Autodesk Fusion 360 part; units mm, degrees
(part 10 of 12)
  line L950 (83.2448, 72.1244) -> (83.2448, 77.1244)
  line L951 (83.2448, 77.1244) -> (78.9146, 79.6244)
  line L952 (89.5749, 79.6244) -> (85.2448, 77.1244)
  line L953 (85.2448, 77.1244) -> (85.2448, 72.1244)
  line L954 (85.2448, 72.1244) -> (89.5749, 69.6244)
  line L955 (89.5749, 69.6244) -> (93.905, 72.1244)
  line L956 (93.905, 72.1244) -> (93.905, 77.1244)
  line L957 (93.905, 77.1244) -> (89.5749, 79.6244)
  line L958 (100.2351, 79.6244) -> (95.905, 77.1244)
  line L959 (95.905, 77.1244) -> (95.905, 72.1244)
  line L960 (95.905, 72.1244) -> (100.2351, 69.6244)
  line L961 (100.2351, 69.6244) -> (104.5653, 72.1244)
  line L962 (104.5653, 72.1244) -> (104.5653, 77.1244)
  line L963 (104.5653, 77.1244) -> (100.2351, 79.6244)
  line L964 (110.8954, 79.6244) -> (106.5653, 77.1244)
  line L965 (106.5653, 77.1244) -> (106.5653, 72.1244)
  line L966 (106.5653, 72.1244) -> (110.8954, 69.6244)
  line L967 (110.8954, 69.6244) -> (115.2255, 72.1244)
  line L968 (115.2255, 72.1244) -> (115.2255, 77.1244)
  line L969 (115.2255, 77.1244) -> (110.8954, 79.6244)
  line L970 (121.5556, 79.6244) -> (117.2255, 77.1244)
  line L971 (117.2255, 77.1244) -> (117.2255, 72.1244)
  line L972 (117.2255, 72.1244) -> (121.5556, 69.6244)
  line L973 (121.5556, 69.6244) -> (125.8858, 72.1244)
  line L974 (125.8858, 72.1244) -> (125.8858, 77.1244)
  line L975 (125.8858, 77.1244) -> (121.5556, 79.6244)
  line L976 (132.2159, 79.6244) -> (127.8858, 77.1244)
  line L977 (127.8858, 77.1244) -> (127.8858, 72.1244)
  line L978 (127.8858, 72.1244) -> (132.2159, 69.6244)
  line L979 (132.2159, 69.6244) -> (136.546, 72.1244)
  line L980 (136.546, 72.1244) -> (136.546, 77.1244)
  line L981 (136.546, 77.1244) -> (132.2159, 79.6244)
  line L982 (142.8762, 79.6244) -> (138.546, 77.1244)
  line L983 (138.546, 77.1244) -> (138.546, 72.1244)
  line L984 (138.546, 72.1244) -> (142.8762, 69.6244)
  line L985 (142.8762, 69.6244) -> (147.2063, 72.1244)
  line L986 (147.2063, 72.1244) -> (147.2063, 77.1244)
  line L987 (147.2063, 77.1244) -> (142.8762, 79.6244)
  line L988 (-64.9988, 88.8564) -> (-69.3289, 86.3564)
  line L989 (-69.3289, 86.3564) -> (-69.3289, 81.3564)
  line L990 (-69.3289, 81.3564) -> (-64.9988, 78.8564)
  line L991 (-64.9988, 78.8564) -> (-60.6687, 81.3564)
  line L992 (-60.6687, 81.3564) -> (-60.6687, 86.3564)
  line L993 (-60.6687, 86.3564) -> (-64.9988, 88.8564)
  line L994 (-54.3385, 88.8564) -> (-58.6687, 86.3564)
  line L995 (-58.6687, 86.3564) -> (-58.6687, 81.3564)
  line L996 (-58.6687, 81.3564) -> (-54.3385, 78.8564)
  line L997 (-54.3385, 78.8564) -> (-50.0084, 81.3564)
  line L998 (-50.0084, 81.3564) -> (-50.0084, 86.3564)
  line L999 (-50.0084, 86.3564) -> (-54.3385, 88.8564)
  line L1000 (-43.6783, 88.8564) -> (-48.0084, 86.3564)
  line L1001 (-48.0084, 86.3564) -> (-48.0084, 81.3564)
  line L1002 (-48.0084, 81.3564) -> (-43.6783, 78.8564)
  line L1003 (-43.6783, 78.8564) -> (-39.3482, 81.3564)
  line L1004 (-39.3482, 81.3564) -> (-39.3482, 86.3564)
  line L1005 (-39.3482, 86.3564) -> (-43.6783, 88.8564)
  line L1006 (-33.018, 88.8564) -> (-37.3482, 86.3564)
  line L1007 (-37.3482, 86.3564) -> (-37.3482, 81.3564)
  line L1008 (-37.3482, 81.3564) -> (-33.018, 78.8564)
  line L1009 (-33.018, 78.8564) -> (-28.6879, 81.3564)
  line L1010 (-28.6879, 81.3564) -> (-28.6879, 86.3564)
  line L1011 (-28.6879, 86.3564) -> (-33.018, 88.8564)
  line L1012 (-22.3578, 88.8564) -> (-26.6879, 86.3564)
  line L1013 (-26.6879, 86.3564) -> (-26.6879, 81.3564)
  line L1014 (-26.6879, 81.3564) -> (-22.3578, 78.8564)
  line L1015 (-22.3578, 78.8564) -> (-18.0277, 81.3564)
  line L1016 (-18.0277, 81.3564) -> (-18.0277, 86.3564)
  line L1017 (-18.0277, 86.3564) -> (-22.3578, 88.8564)
  line L1018 (-11.6975, 88.8564) -> (-16.0277, 86.3564)
  line L1019 (-16.0277, 86.3564) -> (-16.0277, 81.3564)
  line L1020 (-16.0277, 81.3564) -> (-11.6975, 78.8564)
  line L1021 (-11.6975, 78.8564) -> (-7.3674, 81.3564)
  line L1022 (-7.3674, 81.3564) -> (-7.3674, 86.3564)
  line L1023 (-7.3674, 86.3564) -> (-11.6975, 88.8564)
  line L1024 (-1.0373, 88.8564) -> (-5.3674, 86.3564)
  line L1025 (-5.3674, 86.3564) -> (-5.3674, 81.3564)
  line L1026 (-5.3674, 81.3564) -> (-1.0373, 78.8564)
  line L1027 (-1.0373, 78.8564) -> (3.2929, 81.3564)
  line L1028 (3.2929, 81.3564) -> (3.2929, 86.3564)
  line L1029 (3.2929, 86.3564) -> (-1.0373, 88.8564)
  line L1030 (9.623, 88.8564) -> (5.2929, 86.3564)
  line L1031 (5.2929, 86.3564) -> (5.2929, 81.3564)
  line L1032 (5.2929, 81.3564) -> (9.623, 78.8564)
  line L1033 (9.623, 78.8564) -> (13.9531, 81.3564)
  line L1034 (13.9531, 81.3564) -> (13.9531, 86.3564)
  line L1035 (13.9531, 86.3564) -> (9.623, 88.8564)
  line L1036 (20.2832, 88.8564) -> (15.9531, 86.3564)
  line L1037 (15.9531, 86.3564) -> (15.9531, 81.3564)
  line L1038 (15.9531, 81.3564) -> (20.2832, 78.8564)
  line L1039 (20.2832, 78.8564) -> (24.6134, 81.3564)
  line L1040 (24.6134, 81.3564) -> (24.6134, 86.3564)
  line L1041 (24.6134, 86.3564) -> (20.2832, 88.8564)
  line L1042 (30.9435, 88.8564) -> (26.6134, 86.3564)
  line L1043 (26.6134, 86.3564) -> (26.6134, 81.3564)
  line L1044 (26.6134, 81.3564) -> (30.9435, 78.8564)
  line L1045 (30.9435, 78.8564) -> (35.2736, 81.3564)
  line L1046 (35.2736, 81.3564) -> (35.2736, 86.3564)
  line L1047 (35.2736, 86.3564) -> (30.9435, 88.8564)
  line L1048 (41.6037, 88.8564) -> (37.2736, 86.3564)
  line L1049 (37.2736, 86.3564) -> (37.2736, 81.3564)
  line L1050 (37.2736, 81.3564) -> (41.6037, 78.8564)
  line L1051 (41.6037, 78.8564) -> (45.9339, 81.3564)
  line L1052 (45.9339, 81.3564) -> (45.9339, 86.3564)
  line L1053 (45.9339, 86.3564) -> (41.6037, 88.8564)
  line L1054 (52.264, 88.8564) -> (47.9339, 86.3564)
  line L1055 (47.9339, 86.3564) -> (47.9339, 81.3564)
  line L1056 (47.9339, 81.3564) -> (52.264, 78.8564)
  line L1057 (52.264, 78.8564) -> (56.5941, 81.3564)
  line L1058 (56.5941, 81.3564) -> (56.5941, 86.3564)
  line L1059 (56.5941, 86.3564) -> (52.264, 88.8564)
  line L1060 (62.9242, 88.8564) -> (58.5941, 86.3564)
  line L1061 (58.5941, 86.3564) -> (58.5941, 81.3564)
  line L1062 (58.5941, 81.3564) -> (62.9242, 78.8564)
  line L1063 (62.9242, 78.8564) -> (67.2544, 81.3564)
  line L1064 (67.2544, 81.3564) -> (67.2544, 86.3564)
  line L1065 (67.2544, 86.3564) -> (62.9242, 88.8564)
  line L1066 (73.5845, 88.8564) -> (69.2544, 86.3564)
  line L1067 (69.2544, 86.3564) -> (69.2544, 81.3564)
  line L1068 (69.2544, 81.3564) -> (73.5845, 78.8564)
  line L1069 (73.5845, 78.8564) -> (77.9146, 81.3564)
  line L1070 (77.9146, 81.3564) -> (77.9146, 86.3564)
  line L1071 (77.9146, 86.3564) -> (73.5845, 88.8564)
  line L1072 (84.2448, 88.8564) -> (79.9146, 86.3564)
  line L1073 (79.9146, 86.3564) -> (79.9146, 81.3564)
  line L1074 (79.9146, 81.3564) -> (84.2448, 78.8564)
  line L1075 (84.2448, 78.8564) -> (88.5749, 81.3564)
  line L1076 (88.5749, 81.3564) -> (88.5749, 86.3564)
  line L1077 (88.5749, 86.3564) -> (84.2448, 88.8564)
  line L1078 (94.905, 88.8564) -> (90.5749, 86.3564)
  line L1079 (90.5749, 86.3564) -> (90.5749, 81.3564)
  line L1080 (90.5749, 81.3564) -> (94.905, 78.8564)
  line L1081 (94.905, 78.8564) -> (99.2351, 81.3564)
  line L1082 (99.2351, 81.3564) -> (99.2351, 86.3564)
  line L1083 (99.2351, 86.3564) -> (94.905, 88.8564)
  line L1084 (105.5653, 88.8564) -> (101.2351, 86.3564)
  line L1085 (101.2351, 86.3564) -> (101.2351, 81.3564)
  line L1086 (101.2351, 81.3564) -> (105.5653, 78.8564)
  line L1087 (105.5653, 78.8564) -> (109.8954, 81.3564)
  line L1088 (109.8954, 81.3564) -> (109.8954, 86.3564)
  line L1089 (109.8954, 86.3564) -> (105.5653, 88.8564)
  line L1090 (116.2255, 88.8564) -> (111.8954, 86.3564)
  line L1091 (111.8954, 86.3564) -> (111.8954, 81.3564)
  line L1092 (111.8954, 81.3564) -> (116.2255, 78.8564)
  line L1093 (116.2255, 78.8564) -> (120.5556, 81.3564)
  line L1094 (120.5556, 81.3564) -> (120.5556, 86.3564)
  line L1095 (120.5556, 86.3564) -> (116.2255, 88.8564)
  line L1096 (126.8858, 88.8564) -> (122.5556, 86.3564)
  line L1097 (122.5556, 86.3564) -> (122.5556, 81.3564)
  line L1098 (122.5556, 81.3564) -> (126.8858, 78.8564)
  line L1099 (126.8858, 78.8564) -> (131.2159, 81.3564)
  line L1100 (131.2159, 81.3564) -> (131.2159, 86.3564)
  line L1101 (131.2159, 86.3564) -> (126.8858, 88.8564)
  line L1102 (137.546, 88.8564) -> (133.2159, 86.3564)
  line L1103 (133.2159, 86.3564) -> (133.2159, 81.3564)
  line L1104 (133.2159, 81.3564) -> (137.546, 78.8564)
  line L1105 (137.546, 78.8564) -> (141.8762, 81.3564)
  line L1106 (141.8762, 81.3564) -> (141.8762, 86.3564)
  line L1107 (141.8762, 86.3564) -> (137.546, 88.8564)
  line L1108 (148.2063, 88.8564) -> (143.8762, 86.3564)
  line L1109 (143.8762, 86.3564) -> (143.8762, 81.3564)
  line L1110 (143.8762, 81.3564) -> (148.2063, 78.8564)
  line L1111 (148.2063, 78.8564) -> (152.5364, 81.3564)
  line L1112 (152.5364, 81.3564) -> (152.5364, 86.3564)
  line L1113 (152.5364, 86.3564) -> (148.2063, 88.8564)
  line L1114 (-59.6687, 98.0885) -> (-63.9988, 95.5885)
  line L1115 (-63.9988, 95.5885) -> (-63.9988, 90.5885)
  line L1116 (-63.9988, 90.5885) -> (-59.6687, 88.0885)
  line L1117 (-59.6687, 88.0885) -> (-55.3385, 90.5885)
  line L1118 (-55.3385, 90.5885) -> (-55.3385, 95.5885)
  line L1119 (-55.3385, 95.5885) -> (-59.6687, 98.0885)
  line L1120 (-49.0084, 98.0885) -> (-53.3385, 95.5885)
  line L1121 (-53.3385, 95.5885) -> (-53.3385, 90.5885)
  line L1122 (-53.3385, 90.5885) -> (-49.0084, 88.0885)
  line L1123 (-49.0084, 88.0885) -> (-44.6783, 90.5885)
  line L1124 (-44.6783, 90.5885) -> (-44.6783, 95.5885)
  line L1125 (-44.6783, 95.5885) -> (-49.0084, 98.0885)
  line L1126 (-38.3482, 98.0885) -> (-42.6783, 95.5885)
  line L1127 (-42.6783, 95.5885) -> (-42.6783, 90.5885)
  line L1128 (-42.6783, 90.5885) -> (-38.3482, 88.0885)
  line L1129 (-38.3482, 88.0885) -> (-34.018, 90.5885)
  line L1130 (-34.018, 90.5885) -> (-34.018, 95.5885)
  line L1131 (-34.018, 95.5885) -> (-38.3482, 98.0885)
  line L1132 (-27.6879, 98.0885) -> (-32.018, 95.5885)
  line L1133 (-32.018, 95.5885) -> (-32.018, 90.5885)
  line L1134 (-32.018, 90.5885) -> (-27.6879, 88.0885)
  line L1135 (-27.6879, 88.0885) -> (-23.3578, 90.5885)
  line L1136 (-23.3578, 90.5885) -> (-23.3578, 95.5885)
  line L1137 (-23.3578, 95.5885) -> (-27.6879, 98.0885)
  line L1138 (-17.0277, 98.0885) -> (-21.3578, 95.5885)
  line L1139 (-21.3578, 95.5885) -> (-21.3578, 90.5885)
  line L1140 (-21.3578, 90.5885) -> (-17.0277, 88.0885)
  line L1141 (-17.0277, 88.0885) -> (-12.6975, 90.5885)
  line L1142 (-12.6975, 90.5885) -> (-12.6975, 95.5885)
  line L1143 (-12.6975, 95.5885) -> (-17.0277, 98.0885)
  line L1144 (-6.3674, 98.0885) -> (-10.6975, 95.5885)
  line L1145 (-10.6975, 95.5885) -> (-10.6975, 90.5885)
  line L1146 (-10.6975, 90.5885) -> (-6.3674, 88.0885)
  line L1147 (-6.3674, 88.0885) -> (-2.0373, 90.5885)
  line L1148 (-2.0373, 90.5885) -> (-2.0373, 95.5885)
  line L1149 (-2.0373, 95.5885) -> (-6.3674, 98.0885)
  line L1150 (4.2929, 98.0885) -> (-0.0373, 95.5885)
  line L1151 (-0.0373, 95.5885) -> (-0.0373, 90.5885)
  line L1152 (-0.0373, 90.5885) -> (4.2929, 88.0885)
  line L1153 (4.2929, 88.0885) -> (8.623, 90.5885)
  line L1154 (8.623, 90.5885) -> (8.623, 95.5885)
  line L1155 (8.623, 95.5885) -> (4.2929, 98.0885)
  line L1156 (14.9531, 98.0885) -> (10.623, 95.5885)
  line L1157 (10.623, 95.5885) -> (10.623, 90.5885)
  line L1158 (10.623, 90.5885) -> (14.9531, 88.0885)
  line L1159 (14.9531, 88.0885) -> (19.2832, 90.5885)
  line L1160 (19.2832, 90.5885) -> (19.2832, 95.5885)
  line L1161 (19.2832, 95.5885) -> (14.9531, 98.0885)
  line L1162 (25.6134, 98.0885) -> (21.2832, 95.5885)
  line L1163 (21.2832, 95.5885) -> (21.2832, 90.5885)
  line L1164 (21.2832, 90.5885) -> (25.6134, 88.0885)
  line L1165 (25.6134, 88.0885) -> (29.9435, 90.5885)
  line L1166 (29.9435, 90.5885) -> (29.9435, 95.5885)
  line L1167 (29.9435, 95.5885) -> (25.6134, 98.0885)
  line L1168 (36.2736, 98.0885) -> (31.9435, 95.5885)
  line L1169 (31.9435, 95.5885) -> (31.9435, 90.5885)
  line L1170 (31.9435, 90.5885) -> (36.2736, 88.0885)
  line L1171 (36.2736, 88.0885) -> (40.6037, 90.5885)
  line L1172 (40.6037, 90.5885) -> (40.6037, 95.5885)
  line L1173 (40.6037, 95.5885) -> (36.2736, 98.0885)
  line L1174 (46.9339, 98.0885) -> (42.6037, 95.5885)
  line L1175 (42.6037, 95.5885) -> (42.6037, 90.5885)
  line L1176 (42.6037, 90.5885) -> (46.9339, 88.0885)
  line L1177 (46.9339, 88.0885) -> (51.264, 90.5885)
  line L1178 (51.264, 90.5885) -> (51.264, 95.5885)
  line L1179 (51.264, 95.5885) -> (46.9339, 98.0885)
  line L1180 (57.5941, 98.0885) -> (53.264, 95.5885)
  line L1181 (53.264, 95.5885) -> (53.264, 90.5885)
  line L1182 (53.264, 90.5885) -> (57.5941, 88.0885)
  line L1183 (57.5941, 88.0885) -> (61.9242, 90.5885)
  line L1184 (61.9242, 90.5885) -> (61.9242, 95.5885)
  line L1185 (61.9242, 95.5885) -> (57.5941, 98.0885)
  line L1186 (68.2544, 98.0885) -> (63.9242, 95.5885)
  line L1187 (63.9242, 95.5885) -> (63.9242, 90.5885)
  line L1188 (63.9242, 90.5885) -> (68.2544, 88.0885)
  line L1189 (68.2544, 88.0885) -> (72.5845, 90.5885)
  line L1190 (72.5845, 90.5885) -> (72.5845, 95.5885)
  line L1191 (72.5845, 95.5885) -> (68.2544, 98.0885)
  line L1192 (78.9146, 98.0885) -> (74.5845, 95.5885)
  line L1193 (74.5845, 95.5885) -> (74.5845, 90.5885)
  line L1194 (74.5845, 90.5885) -> (78.9146, 88.0885)
  line L1195 (78.9146, 88.0885) -> (83.2448, 90.5885)
  line L1196 (83.2448, 90.5885) -> (83.2448, 95.5885)
  line L1197 (83.2448, 95.5885) -> (78.9146, 98.0885)
  line L1198 (89.5749, 98.0885) -> (85.2448, 95.5885)
  line L1199 (85.2448, 95.5885) -> (85.2448, 90.5885)
  line L1200 (85.2448, 90.5885) -> (89.5749, 88.0885)
  line L1201 (89.5749, 88.0885) -> (93.905, 90.5885)
  line L1202 (93.905, 90.5885) -> (93.905, 95.5885)
  line L1203 (93.905, 95.5885) -> (89.5749, 98.0885)
  line L1204 (100.2351, 98.0885) -> (95.905, 95.5885)
  line L1205 (95.905, 95.5885) -> (95.905, 90.5885)
  line L1206 (95.905, 90.5885) -> (100.2351, 88.0885)
  line L1207 (100.2351, 88.0885) -> (104.5653, 90.5885)
  line L1208 (104.5653, 90.5885) -> (104.5653, 95.5885)
  line L1209 (104.5653, 95.5885) -> (100.2351, 98.0885)
  line L1210 (110.8954, 98.0885) -> (106.5653, 95.5885)
  line L1211 (106.5653, 95.5885) -> (106.5653, 90.5885)
  line L1212 (106.5653, 90.5885) -> (110.8954, 88.0885)
  line L1213 (110.8954, 88.0885) -> (115.2255, 90.5885)
  line L1214 (115.2255, 90.5885) -> (115.2255, 95.5885)
  line L1215 (115.2255, 95.5885) -> (110.8954, 98.0885)
  line L1216 (121.5556, 98.0885) -> (117.2255, 95.5885)
  line L1217 (117.2255, 95.5885) -> (117.2255, 90.5885)
  line L1218 (117.2255, 90.5885) -> (121.5556, 88.0885)
  line L1219 (121.5556, 88.0885) -> (125.8858, 90.5885)
  line L1220 (125.8858, 90.5885) -> (125.8858, 95.5885)
  line L1221 (125.8858, 95.5885) -> (121.5556, 98.0885)
  line L1222 (132.2159, 98.0885) -> (127.8858, 95.5885)
  line L1223 (127.8858, 95.5885) -> (127.8858, 90.5885)
  line L1224 (127.8858, 90.5885) -> (132.2159, 88.0885)
  line L1225 (132.2159, 88.0885) -> (136.546, 90.5885)
  line L1226 (136.546, 90.5885) -> (136.546, 95.5885)
  line L1227 (136.546, 95.5885) -> (132.2159, 98.0885)
  line L1228 (142.8762, 98.0885) -> (138.546, 95.5885)
  line L1229 (138.546, 95.5885) -> (138.546, 90.5885)
  line L1230 (138.546, 90.5885) -> (142.8762, 88.0885)
  line L1231 (142.8762, 88.0885) -> (147.2063, 90.5885)
  line L1232 (147.2063, 90.5885) -> (147.2063, 95.5885)
  line L1233 (147.2063, 95.5885) -> (142.8762, 98.0885)
  line L1234 (-64.9988, 107.3205) -> (-69.3289, 104.8205)
  line L1235 (-69.3289, 104.8205) -> (-69.3289, 99.8205)
  line L1236 (-69.3289, 99.8205) -> (-64.9988, 97.3205)
  line L1237 (-64.9988, 97.3205) -> (-60.6687, 99.8205)
  line L1238 (-60.6687, 99.8205) -> (-60.6687, 104.8205)
  line L1239 (-60.6687, 104.8205) -> (-64.9988, 107.3205)
  line L1240 (-54.3385, 107.3205) -> (-58.6687, 104.8205)
  line L1241 (-58.6687, 104.8205) -> (-58.6687, 99.8205)
  line L1242 (-58.6687, 99.8205) -> (-54.3385, 97.3205)
  line L1243 (-54.3385, 97.3205) -> (-50.0084, 99.8205)
  line L1244 (-50.0084, 99.8205) -> (-50.0084, 104.8205)
  line L1245 (-50.0084, 104.8205) -> (-54.3385, 107.3205)
  line L1246 (-43.6783, 107.3205) -> (-48.0084, 104.8205)
  line L1247 (-48.0084, 104.8205) -> (-48.0084, 99.8205)
  line L1248 (-48.0084, 99.8205) -> (-43.6783, 97.3205)
  line L1249 (-43.6783, 97.3205) -> (-39.3482, 99.8205)
  line L1250 (-39.3482, 99.8205) -> (-39.3482, 104.8205)
  line L1251 (-39.3482, 104.8205) -> (-43.6783, 107.3205)
  line L1252 (-33.018, 107.3205) -> (-37.3482, 104.8205)
  line L1253 (-37.3482, 104.8205) -> (-37.3482, 99.8205)
  line L1254 (-37.3482, 99.8205) -> (-33.018, 97.3205)
  line L1255 (-33.018, 97.3205) -> (-28.6879, 99.8205)
  line L1256 (-28.6879, 99.8205) -> (-28.6879, 104.8205)
  line L1257 (-28.6879, 104.8205) -> (-33.018, 107.3205)
  line L1258 (-22.3578, 107.3205) -> (-26.6879, 104.8205)
  line L1259 (-26.6879, 104.8205) -> (-26.6879, 99.8205)
  line L1260 (-26.6879, 99.8205) -> (-22.3578, 97.3205)
  line L1261 (-22.3578, 97.3205) -> (-18.0277, 99.8205)
  line L1262 (-18.0277, 99.8205) -> (-18.0277, 104.8205)
  line L1263 (-18.0277, 104.8205) -> (-22.3578, 107.3205)
  line L1264 (-11.6975, 107.3205) -> (-16.0277, 104.8205)
  line L1265 (-16.0277, 104.8205) -> (-16.0277, 99.8205)
  line L1266 (-16.0277, 99.8205) -> (-11.6975, 97.3205)
  line L1267 (-11.6975, 97.3205) -> (-7.3674, 99.8205)
  line L1268 (-7.3674, 99.8205) -> (-7.3674, 104.8205)
  line L1269 (-7.3674, 104.8205) -> (-11.6975, 107.3205)
  line L1270 (-1.0373, 107.3205) -> (-5.3674, 104.8205)
  line L1271 (-5.3674, 104.8205) -> (-5.3674, 99.8205)
  line L1272 (-5.3674, 99.8205) -> (-1.0373, 97.3205)
  line L1273 (-1.0373, 97.3205) -> (3.2929, 99.8205)
  line L1274 (3.2929, 99.8205) -> (3.2929, 104.8205)
  line L1275 (3.2929, 104.8205) -> (-1.0373, 107.3205)
  line L1276 (9.623, 107.3205) -> (5.2929, 104.8205)
  line L1277 (5.2929, 104.8205) -> (5.2929, 99.8205)
  line L1278 (5.2929, 99.8205) -> (9.623, 97.3205)
  line L1279 (9.623, 97.3205) -> (13.9531, 99.8205)
  line L1280 (13.9531, 99.8205) -> (13.9531, 104.8205)
  line L1281 (13.9531, 104.8205) -> (9.623, 107.3205)
  line L1282 (20.2832, 107.3205) -> (15.9531, 104.8205)
  line L1283 (15.9531, 104.8205) -> (15.9531, 99.8205)
  line L1284 (15.9531, 99.8205) -> (20.2832, 97.3205)
  line L1285 (20.2832, 97.3205) -> (24.6134, 99.8205)
  line L1286 (24.6134, 99.8205) -> (24.6134, 104.8205)
  line L1287 (24.6134, 104.8205) -> (20.2832, 107.3205)
  line L1288 (30.9435, 107.3205) -> (26.6134, 104.8205)
  line L1289 (26.6134, 104.8205) -> (26.6134, 99.8205)
  line L1290 (26.6134, 99.8205) -> (30.9435, 97.3205)
  line L1291 (30.9435, 97.3205) -> (35.2736, 99.8205)
  line L1292 (35.2736, 99.8205) -> (35.2736, 104.8205)
  line L1293 (35.2736, 104.8205) -> (30.9435, 107.3205)
  line L1294 (41.6037, 107.3205) -> (37.2736, 104.8205)
  line L1295 (37.2736, 104.8205) -> (37.2736, 99.8205)
  line L1296 (37.2736, 99.8205) -> (41.6037, 97.3205)
  line L1297 (41.6037, 97.3205) -> (45.9339, 99.8205)
  line L1298 (45.9339, 99.8205) -> (45.9339, 104.8205)
  line L1299 (45.9339, 104.8205) -> (41.6037, 107.3205)
  line L1300 (52.264, 107.3205) -> (47.9339, 104.8205)
  line L1301 (47.9339, 104.8205) -> (47.9339, 99.8205)
  line L1302 (47.9339, 99.8205) -> (52.264, 97.3205)
  line L1303 (52.264, 97.3205) -> (56.5941, 99.8205)
  line L1304 (56.5941, 99.8205) -> (56.5941, 104.8205)
  line L1305 (56.5941, 104.8205) -> (52.264, 107.3205)
  line L1306 (62.9242, 107.3205) -> (58.5941, 104.8205)
  line L1307 (58.5941, 104.8205) -> (58.5941, 99.8205)
  line L1308 (58.5941, 99.8205) -> (62.9242, 97.3205)
  line L1309 (62.9242, 97.3205) -> (67.2544, 99.8205)
  line L1310 (67.2544, 99.8205) -> (67.2544, 104.8205)
  line L1311 (67.2544, 104.8205) -> (62.9242, 107.3205)
  line L1312 (73.5845, 107.3205) -> (69.2544, 104.8205)
  line L1313 (69.2544, 104.8205) -> (69.2544, 99.8205)
  line L1314 (69.2544, 99.8205) -> (73.5845, 97.3205)
  line L1315 (73.5845, 97.3205) -> (77.9146, 99.8205)
  line L1316 (77.9146, 99.8205) -> (77.9146, 104.8205)
  line L1317 (77.9146, 104.8205) -> (73.5845, 107.3205)
  line L1318 (84.2448, 107.3205) -> (79.9146, 104.8205)
  line L1319 (79.9146, 104.8205) -> (79.9146, 99.8205)
  line L1320 (79.9146, 99.8205) -> (84.2448, 97.3205)
  line L1321 (84.2448, 97.3205) -> (88.5749, 99.8205)
  line L1322 (88.5749, 99.8205) -> (88.5749, 104.8205)
  line L1323 (88.5749, 104.8205) -> (84.2448, 107.3205)
  line L1324 (94.905, 107.3205) -> (90.5749, 104.8205)
  line L1325 (90.5749, 104.8205) -> (90.5749, 99.8205)
  line L1326 (90.5749, 99.8205) -> (94.905, 97.3205)
  line L1327 (94.905, 97.3205) -> (99.2351, 99.8205)
  line L1328 (99.2351, 99.8205) -> (99.2351, 104.8205)
  line L1329 (99.2351, 104.8205) -> (94.905, 107.3205)
  line L1330 (105.5653, 107.3205) -> (101.2351, 104.8205)
  line L1331 (101.2351, 104.8205) -> (101.2351, 99.8205)
  line L1332 (101.2351, 99.8205) -> (105.5653, 97.3205)
  line L1333 (105.5653, 97.3205) -> (109.8954, 99.8205)
  line L1334 (109.8954, 99.8205) -> (109.8954, 104.8205)
  line L1335 (109.8954, 104.8205) -> (105.5653, 107.3205)
  line L1336 (116.2255, 107.3205) -> (111.8954, 104.8205)
  line L1337 (111.8954, 104.8205) -> (111.8954, 99.8205)
  line L1338 (111.8954, 99.8205) -> (116.2255, 97.3205)
  line L1339 (116.2255, 97.3205) -> (120.5556, 99.8205)
  line L1340 (120.5556, 99.8205) -> (120.5556, 104.8205)
  line L1341 (120.5556, 104.8205) -> (116.2255, 107.3205)
  line L1342 (126.8858, 107.3205) -> (122.5556, 104.8205)
  line L1343 (122.5556, 104.8205) -> (122.5556, 99.8205)
  line L1344 (122.5556, 99.8205) -> (126.8858, 97.3205)
  line L1345 (126.8858, 97.3205) -> (131.2159, 99.8205)
  line L1346 (131.2159, 99.8205) -> (131.2159, 104.8205)
  line L1347 (131.2159, 104.8205) -> (126.8858, 107.3205)
  line L1348 (137.546, 107.3205) -> (133.2159, 104.8205)
  line L1349 (133.2159, 104.8205) -> (133.2159, 99.8205)
  line L1350 (133.2159, 99.8205) -> (137.546, 97.3205)
  line L1351 (137.546, 97.3205) -> (141.8762, 99.8205)
  line L1352 (141.8762, 99.8205) -> (141.8762, 104.8205)
  line L1353 (141.8762, 104.8205) -> (137.546, 107.3205)
  line L1354 (148.2063, 107.3205) -> (143.8762, 104.8205)
  line L1355 (143.8762, 104.8205) -> (143.8762, 99.8205)
  line L1356 (143.8762, 99.8205) -> (148.2063, 97.3205)
  line L1357 (148.2063, 97.3205) -> (152.5364, 99.8205)
  line L1358 (152.5364, 99.8205) -> (152.5364, 104.8205)
  line L1359 (152.5364, 104.8205) -> (148.2063, 107.3205)
  line L1360 (-59.6687, 116.5526) -> (-63.9988, 114.0526)
  line L1361 (-63.9988, 114.0526) -> (-63.9988, 109.0526)
  line L1362 (-63.9988, 109.0526) -> (-59.6687, 106.5526)
  line L1363 (-59.6687, 106.5526) -> (-55.3385, 109.0526)
  line L1364 (-55.3385, 109.0526) -> (-55.3385, 114.0526)
  line L1365 (-55.3385, 114.0526) -> (-59.6687, 116.5526)
  line L1366 (-49.0084, 116.5526) -> (-53.3385, 114.0526)
  line L1367 (-53.3385, 114.0526) -> (-53.3385, 109.0526)
  line L1368 (-53.3385, 109.0526) -> (-49.0084, 106.5526)
  line L1369 (-49.0084, 106.5526) -> (-44.6783, 109.0526)
  line L1370 (-44.6783, 109.0526) -> (-44.6783, 114.0526)
  line L1371 (-44.6783, 114.0526) -> (-49.0084, 116.5526)
  line L1372 (-38.3482, 116.5526) -> (-42.6783, 114.0526)
  line L1373 (-42.6783, 114.0526) -> (-42.6783, 109.0526)
  line L1374 (-42.6783, 109.0526) -> (-38.3482, 106.5526)
  line L1375 (-38.3482, 106.5526) -> (-34.018, 109.0526)
  line L1376 (-34.018, 109.0526) -> (-34.018, 114.0526)
  line L1377 (-34.018, 114.0526) -> (-38.3482, 116.5526)
  line L1378 (-27.6879, 116.5526) -> (-32.018, 114.0526)
  line L1379 (-32.018, 114.0526) -> (-32.018, 109.0526)
  line L1380 (-32.018, 109.0526) -> (-27.6879, 106.5526)
  line L1381 (-27.6879, 106.5526) -> (-23.3578, 109.0526)
  line L1382 (-23.3578, 109.0526) -> (-23.3578, 114.0526)
  line L1383 (-23.3578, 114.0526) -> (-27.6879, 116.5526)
  line L1384 (-17.0277, 116.5526) -> (-21.3578, 114.0526)
  line L1385 (-21.3578, 114.0526) -> (-21.3578, 109.0526)
  line L1386 (-21.3578, 109.0526) -> (-17.0277, 106.5526)
  line L1387 (-17.0277, 106.5526) -> (-12.6975, 109.0526)
  line L1388 (-12.6975, 109.0526) -> (-12.6975, 114.0526)
  line L1389 (-12.6975, 114.0526) -> (-17.0277, 116.5526)
  line L1390 (-6.3674, 116.5526) -> (-10.6975, 114.0526)
  line L1391 (-10.6975, 114.0526) -> (-10.6975, 109.0526)
  line L1392 (-10.6975, 109.0526) -> (-6.3674, 106.5526)
  line L1393 (-6.3674, 106.5526) -> (-2.0373, 109.0526)
  line L1394 (-2.0373, 109.0526) -> (-2.0373, 114.0526)
  line L1395 (-2.0373, 114.0526) -> (-6.3674, 116.5526)
  line L1396 (4.2929, 116.5526) -> (-0.0373, 114.0526)
  line L1397 (-0.0373, 114.0526) -> (-0.0373, 109.0526)
  line L1398 (-0.0373, 109.0526) -> (4.2929, 106.5526)
  line L1399 (4.2929, 106.5526) -> (8.623, 109.0526)
  line L1400 (8.623, 109.0526) -> (8.623, 114.0526)
  line L1401 (8.623, 114.0526) -> (4.2929, 116.5526)
  line L1402 (14.9531, 116.5526) -> (10.623, 114.0526)
  line L1403 (10.623, 114.0526) -> (10.623, 109.0526)
  line L1404 (10.623, 109.0526) -> (14.9531, 106.5526)
  line L1405 (14.9531, 106.5526) -> (19.2832, 109.0526)
  line L1406 (19.2832, 109.0526) -> (19.2832, 114.0526)
  line L1407 (19.2832, 114.0526) -> (14.9531, 116.5526)
  line L1408 (25.6134, 116.5526) -> (21.2832, 114.0526)
  line L1409 (21.2832, 114.0526) -> (21.2832, 109.0526)
  line L1410 (21.2832, 109.0526) -> (25.6134, 106.5526)
  line L1411 (25.6134, 106.5526) -> (29.9435, 109.0526)
  line L1412 (29.9435, 109.0526) -> (29.9435, 114.0526)
  line L1413 (29.9435, 114.0526) -> (25.6134, 116.5526)
  line L1414 (36.2736, 116.5526) -> (31.9435, 114.0526)
  line L1415 (31.9435, 114.0526) -> (31.9435, 109.0526)
  line L1416 (31.9435, 109.0526) -> (36.2736, 106.5526)
  line L1417 (36.2736, 106.5526) -> (40.6037, 109.0526)
  line L1418 (40.6037, 109.0526) -> (40.6037, 114.0526)
  line L1419 (40.6037, 114.0526) -> (36.2736, 116.5526)
  line L1420 (46.9339, 116.5526) -> (42.6037, 114.0526)
  line L1421 (42.6037, 114.0526) -> (42.6037, 109.0526)
  line L1422 (42.6037, 109.0526) -> (46.9339, 106.5526)
  line L1423 (46.9339, 106.5526) -> (51.264, 109.0526)
  line L1424 (51.264, 109.0526) -> (51.264, 114.0526)
  line L1425 (51.264, 114.0526) -> (46.9339, 116.5526)
  line L1426 (57.5941, 116.5526) -> (53.264, 114.0526)
  line L1427 (53.264, 114.0526) -> (53.264, 109.0526)
  line L1428 (53.264, 109.0526) -> (57.5941, 106.5526)
  line L1429 (57.5941, 106.5526) -> (61.9242, 109.0526)
  line L1430 (61.9242, 109.0526) -> (61.9242, 114.0526)
  line L1431 (61.9242, 114.0526) -> (57.5941, 116.5526)
  line L1432 (68.2544, 116.5526) -> (63.9242, 114.0526)
  line L1433 (63.9242, 114.0526) -> (63.9242, 109.0526)
  line L1434 (63.9242, 109.0526) -> (68.2544, 106.5526)
  line L1435 (68.2544, 106.5526) -> (72.5845, 109.0526)
  line L1436 (72.5845, 109.0526) -> (72.5845, 114.0526)
  line L1437 (72.5845, 114.0526) -> (68.2544, 116.5526)
  line L1438 (78.9146, 116.5526) -> (74.5845, 114.0526)
  line L1439 (74.5845, 114.0526) -> (74.5845, 109.0526)
  line L1440 (74.5845, 109.0526) -> (78.9146, 106.5526)
  line L1441 (78.9146, 106.5526) -> (83.2448, 109.0526)
  line L1442 (83.2448, 109.0526) -> (83.2448, 114.0526)
  line L1443 (83.2448, 114.0526) -> (78.9146, 116.5526)
  line L1444 (89.5749, 116.5526) -> (85.2448, 114.0526)
  line L1445 (85.2448, 114.0526) -> (85.2448, 109.0526)
  line L1446 (85.2448, 109.0526) -> (89.5749, 106.5526)
  line L1447 (89.5749, 106.5526) -> (93.905, 109.0526)
  line L1448 (93.905, 109.0526) -> (93.905, 114.0526)
  line L1449 (93.905, 114.0526) -> (89.5749, 116.5526)
  line L1450 (100.2351, 116.5526) -> (95.905, 114.0526)
  line L1451 (95.905, 114.0526) -> (95.905, 109.0526)
  line L1452 (95.905, 109.0526) -> (100.2351, 106.5526)
  line L1453 (100.2351, 106.5526) -> (104.5653, 109.0526)
  line L1454 (104.5653, 109.0526) -> (104.5653, 114.0526)
  line L1455 (104.5653, 114.0526) -> (100.2351, 116.5526)
  line L1456 (110.8954, 116.5526) -> (106.5653, 114.0526)
  line L1457 (106.5653, 114.0526) -> (106.5653, 109.0526)
  line L1458 (106.5653, 109.0526) -> (110.8954, 106.5526)
  line L1459 (110.8954, 106.5526) -> (115.2255, 109.0526)
  line L1460 (115.2255, 109.0526) -> (115.2255, 114.0526)
  line L1461 (115.2255, 114.0526) -> (110.8954, 116.5526)
  line L1462 (121.5556, 116.5526) -> (117.2255, 114.0526)
  line L1463 (117.2255, 114.0526) -> (117.2255, 109.0526)
  line L1464 (117.2255, 109.0526) -> (121.5556, 106.5526)
  line L1465 (121.5556, 106.5526) -> (125.8858, 109.0526)
  line L1466 (125.8858, 109.0526) -> (125.8858, 114.0526)
  line L1467 (125.8858, 114.0526) -> (121.5556, 116.5526)
  line L1468 (132.2159, 116.5526) -> (127.8858, 114.0526)
  line L1469 (127.8858, 114.0526) -> (127.8858, 109.0526)
  line L1470 (127.8858, 109.0526) -> (132.2159, 106.5526)
  line L1471 (132.2159, 106.5526) -> (136.546, 109.0526)
  line L1472 (136.546, 109.0526) -> (136.546, 114.0526)
  line L1473 (136.546, 114.0526) -> (132.2159, 116.5526)
  line L1474 (142.8762, 116.5526) -> (138.546, 114.0526)
  line L1475 (138.546, 114.0526) -> (138.546, 109.0526)
  line L1476 (138.546, 109.0526) -> (142.8762, 106.5526)
  line L1477 (142.8762, 106.5526) -> (147.2063, 109.0526)
  line L1478 (147.2063, 109.0526) -> (147.2063, 114.0526)
  line L1479 (147.2063, 114.0526) -> (142.8762, 116.5526)
  line L1480 (-64.9988, 125.7846) -> (-69.3289, 123.2846)
  line L1481 (-69.3289, 123.2846) -> (-69.3289, 118.2846)
  line L1482 (-69.3289, 118.2846) -> (-64.9988, 115.7846)
  line L1483 (-64.9988, 115.7846) -> (-60.6687, 118.2846)
  line L1484 (-60.6687, 118.2846) -> (-60.6687, 123.2846)
  line L1485 (-60.6687, 123.2846) -> (-64.9988, 125.7846)
  line L1486 (-54.3385, 125.7846) -> (-58.6687, 123.2846)
  line L1487 (-58.6687, 123.2846) -> (-58.6687, 118.2846)
  line L1488 (-58.6687, 118.2846) -> (-54.3385, 115.7846)
  line L1489 (-54.3385, 115.7846) -> (-50.0084, 118.2846)
  line L1490 (-50.0084, 118.2846) -> (-50.0084, 123.2846)
  line L1491 (-50.0084, 123.2846) -> (-54.3385, 125.7846)
  line L1492 (-43.6783, 125.7846) -> (-48.0084, 123.2846)
  line L1493 (-48.0084, 123.2846) -> (-48.0084, 118.2846)
  line L1494 (-48.0084, 118.2846) -> (-43.6783, 115.7846)
  line L1495 (-43.6783, 115.7846) -> (-39.3482, 118.2846)
  line L1496 (-39.3482, 118.2846) -> (-39.3482, 123.2846)
  line L1497 (-39.3482, 123.2846) -> (-43.6783, 125.7846)
  line L1498 (-33.018, 125.7846) -> (-37.3482, 123.2846)
  line L1499 (-37.3482, 123.2846) -> (-37.3482, 118.2846)
  line L1500 (-37.3482, 118.2846) -> (-33.018, 115.7846)
  line L1501 (-33.018, 115.7846) -> (-28.6879, 118.2846)
  line L1502 (-28.6879, 118.2846) -> (-28.6879, 123.2846)
  line L1503 (-28.6879, 123.2846) -> (-33.018, 125.7846)
  line L1504 (-22.3578, 125.7846) -> (-26.6879, 123.2846)
  line L1505 (-26.6879, 123.2846) -> (-26.6879, 118.2846)
  line L1506 (-26.6879, 118.2846) -> (-22.3578, 115.7846)
  line L1507 (-22.3578, 115.7846) -> (-18.0277, 118.2846)
  line L1508 (-18.0277, 118.2846) -> (-18.0277, 123.2846)
  line L1509 (-18.0277, 123.2846) -> (-22.3578, 125.7846)
  line L1510 (-11.6975, 125.7846) -> (-16.0277, 123.2846)
  line L1511 (-16.0277, 123.2846) -> (-16.0277, 118.2846)
  line L1512 (-16.0277, 118.2846) -> (-11.6975, 115.7846)
  line L1513 (-11.6975, 115.7846) -> (-7.3674, 118.2846)
  line L1514 (-7.3674, 118.2846) -> (-7.3674, 123.2846)
  line L1515 (-7.3674, 123.2846) -> (-11.6975, 125.7846)
  line L1516 (-1.0373, 125.7846) -> (-5.3674, 123.2846)
  line L1517 (-5.3674, 123.2846) -> (-5.3674, 118.2846)
  line L1518 (-5.3674, 118.2846) -> (-1.0373, 115.7846)
  line L1519 (-1.0373, 115.7846) -> (3.2929, 118.2846)
  line L1520 (3.2929, 118.2846) -> (3.2929, 123.2846)
  line L1521 (3.2929, 123.2846) -> (-1.0373, 125.7846)
  line L1522 (9.623, 125.7846) -> (5.2929, 123.2846)
  line L1523 (5.2929, 123.2846) -> (5.2929, 118.2846)
  line L1524 (5.2929, 118.2846) -> (9.623, 115.7846)
  line L1525 (9.623, 115.7846) -> (13.9531, 118.2846)
  line L1526 (13.9531, 118.2846) -> (13.9531, 123.2846)
  line L1527 (13.9531, 123.2846) -> (9.623, 125.7846)
  line L1528 (20.2832, 125.7846) -> (15.9531, 123.2846)
  line L1529 (15.9531, 123.2846) -> (15.9531, 118.2846)
  line L1530 (15.9531, 118.2846) -> (20.2832, 115.7846)
  line L1531 (20.2832, 115.7846) -> (24.6134, 118.2846)
  line L1532 (24.6134, 118.2846) -> (24.6134, 123.2846)
  line L1533 (24.6134, 123.2846) -> (20.2832, 125.7846)
  line L1534 (30.9435, 125.7846) -> (26.6134, 123.2846)
  line L1535 (26.6134, 123.2846) -> (26.6134, 118.2846)
  line L1536 (26.6134, 118.2846) -> (30.9435, 115.7846)
  line L1537 (30.9435, 115.7846) -> (35.2736, 118.2846)
  line L1538 (35.2736, 118.2846) -> (35.2736, 123.2846)
  line L1539 (35.2736, 123.2846) -> (30.9435, 125.7846)
  line L1540 (41.6037, 125.7846) -> (37.2736, 123.2846)
  line L1541 (37.2736, 123.2846) -> (37.2736, 118.2846)
  line L1542 (37.2736, 118.2846) -> (41.6037, 115.7846)
  line L1543 (41.6037, 115.7846) -> (45.9339, 118.2846)
  line L1544 (45.9339, 118.2846) -> (45.9339, 123.2846)
  line L1545 (45.9339, 123.2846) -> (41.6037, 125.7846)
  line L1546 (52.264, 125.7846) -> (47.9339, 123.2846)
  line L1547 (47.9339, 123.2846) -> (47.9339, 118.2846)
  line L1548 (47.9339, 118.2846) -> (52.264, 115.7846)
  line L1549 (52.264, 115.7846) -> (56.5941, 118.2846)
  line L1550 (56.5941, 118.2846) -> (56.5941, 123.2846)
  line L1551 (56.5941, 123.2846) -> (52.264, 125.7846)
  line L1552 (62.9242, 125.7846) -> (58.5941, 123.2846)
  line L1553 (58.5941, 123.2846) -> (58.5941, 118.2846)
  line L1554 (58.5941, 118.2846) -> (62.9242, 115.7846)
  line L1555 (62.9242, 115.7846) -> (67.2544, 118.2846)
  line L1556 (67.2544, 118.2846) -> (67.2544, 123.2846)
  line L1557 (67.2544, 123.2846) -> (62.9242, 125.7846)
  line L1558 (73.5845, 125.7846) -> (69.2544, 123.2846)
  line L1559 (69.2544, 123.2846) -> (69.2544, 118.2846)
  line L1560 (69.2544, 118.2846) -> (73.5845, 115.7846)
  line L1561 (73.5845, 115.7846) -> (77.9146, 118.2846)
  line L1562 (77.9146, 118.2846) -> (77.9146, 123.2846)
  line L1563 (77.9146, 123.2846) -> (73.5845, 125.7846)
  line L1564 (84.2448, 125.7846) -> (79.9146, 123.2846)
  line L1565 (79.9146, 123.2846) -> (79.9146, 118.2846)
  line L1566 (79.9146, 118.2846) -> (84.2448, 115.7846)
  line L1567 (84.2448, 115.7846) -> (88.5749, 118.2846)
  line L1568 (88.5749, 118.2846) -> (88.5749, 123.2846)
  line L1569 (88.5749, 123.2846) -> (84.2448, 125.7846)
  line L1570 (94.905, 125.7846) -> (90.5749, 123.2846)
  line L1571 (90.5749, 123.2846) -> (90.5749, 118.2846)
  line L1572 (90.5749, 118.2846) -> (94.905, 115.7846)
  line L1573 (94.905, 115.7846) -> (99.2351, 118.2846)
  line L1574 (99.2351, 118.2846) -> (99.2351, 123.2846)
  line L1575 (99.2351, 123.2846) -> (94.905, 125.7846)
  line L1576 (105.5653, 125.7846) -> (101.2351, 123.2846)
  line L1577 (101.2351, 123.2846) -> (101.2351, 118.2846)
  line L1578 (101.2351, 118.2846) -> (105.5653, 115.7846)
  line L1579 (105.5653, 115.7846) -> (109.8954, 118.2846)
  line L1580 (109.8954, 118.2846) -> (109.8954, 123.2846)
  line L1581 (109.8954, 123.2846) -> (105.5653, 125.7846)
  line L1582 (116.2255, 125.7846) -> (111.8954, 123.2846)
  line L1583 (111.8954, 123.2846) -> (111.8954, 118.2846)
  line L1584 (111.8954, 118.2846) -> (116.2255, 115.7846)
  line L1585 (116.2255, 115.7846) -> (120.5556, 118.2846)
  line L1586 (120.5556, 118.2846) -> (120.5556, 123.2846)
  line L1587 (120.5556, 123.2846) -> (116.2255, 125.7846)
  line L1588 (126.8858, 125.7846) -> (122.5556, 123.2846)
  line L1589 (122.5556, 123.2846) -> (122.5556, 118.2846)
  line L1590 (122.5556, 118.2846) -> (126.8858, 115.7846)
  line L1591 (126.8858, 115.7846) -> (131.2159, 118.2846)
  line L1592 (131.2159, 118.2846) -> (131.2159, 123.2846)
  line L1593 (131.2159, 123.2846) -> (126.8858, 125.7846)
  line L1594 (137.546, 125.7846) -> (133.2159, 123.2846)
  line L1595 (133.2159, 123.2846) -> (133.2159, 118.2846)
  line L1596 (133.2159, 118.2846) -> (137.546, 115.7846)
  line L1597 (137.546, 115.7846) -> (141.8762, 118.2846)
  line L1598 (141.8762, 118.2846) -> (141.8762, 123.2846)
  line L1599 (141.8762, 123.2846) -> (137.546, 125.7846)
  line L1600 (148.2063, 125.7846) -> (143.8762, 123.2846)
  line L1601 (143.8762, 123.2846) -> (143.8762, 118.2846)
  line L1602 (143.8762, 118.2846) -> (148.2063, 115.7846)
  line L1603 (148.2063, 115.7846) -> (152.5364, 118.2846)
  line L1604 (152.5364, 118.2846) -> (152.5364, 123.2846)
  line L1605 (152.5364, 123.2846) -> (148.2063, 125.7846)
  line L1606 (-59.6687, 135.0167) -> (-63.9988, 132.5167)
  line L1607 (-63.9988, 132.5167) -> (-63.9988, 127.5167)
  line L1608 (-63.9988, 127.5167) -> (-59.6687, 125.0167)
  line L1609 (-59.6687, 125.0167) -> (-55.3385, 127.5167)
  line L1610 (-55.3385, 127.5167) -> (-55.3385, 132.5167)
  line L1611 (-55.3385, 132.5167) -> (-59.6687, 135.0167)
  line L1612 (-49.0084, 135.0167) -> (-53.3385, 132.5167)
  line L1613 (-53.3385, 132.5167) -> (-53.3385, 127.5167)
  line L1614 (-53.3385, 127.5167) -> (-49.0084, 125.0167)
  line L1615 (-49.0084, 125.0167) -> (-44.6783, 127.5167)
  line L1616 (-44.6783, 127.5167) -> (-44.6783, 132.5167)
  line L1617 (-44.6783, 132.5167) -> (-49.0084, 135.0167)
  line L1618 (-38.3482, 135.0167) -> (-42.6783, 132.5167)
  line L1619 (-42.6783, 132.5167) -> (-42.6783, 127.5167)
  line L1620 (-42.6783, 127.5167) -> (-38.3482, 125.0167)
  line L1621 (-38.3482, 125.0167) -> (-34.018, 127.5167)
  line L1622 (-34.018, 127.5167) -> (-34.018, 132.5167)
  line L1623 (-34.018, 132.5167) -> (-38.3482, 135.0167)
  line L1624 (-27.6879, 135.0167) -> (-32.018, 132.5167)
  line L1625 (-32.018, 132.5167) -> (-32.018, 127.5167)
  line L1626 (-32.018, 127.5167) -> (-27.6879, 125.0167)
  line L1627 (-27.6879, 125.0167) -> (-23.3578, 127.5167)
  line L1628 (-23.3578, 127.5167) -> (-23.3578, 132.5167)
  line L1629 (-23.3578, 132.5167) -> (-27.6879, 135.0167)
  line L1630 (-17.0277, 135.0167) -> (-21.3578, 132.5167)
  line L1631 (-21.3578, 132.5167) -> (-21.3578, 127.5167)
  line L1632 (-21.3578, 127.5167) -> (-17.0277, 125.0167)
  line L1633 (-17.0277, 125.0167) -> (-12.6975, 127.5167)
  line L1634 (-12.6975, 127.5167) -> (-12.6975, 132.5167)
  line L1635 (-12.6975, 132.5167) -> (-17.0277, 135.0167)
  line L1636 (-6.3674, 135.0167) -> (-10.6975, 132.5167)
  line L1637 (-10.6975, 132.5167) -> (-10.6975, 127.5167)
  line L1638 (-10.6975, 127.5167) -> (-6.3674, 125.0167)
  line L1639 (-6.3674, 125.0167) -> (-2.0373, 127.5167)
  line L1640 (-2.0373, 127.5167) -> (-2.0373, 132.5167)
  line L1641 (-2.0373, 132.5167) -> (-6.3674, 135.0167)
  line L1642 (4.2929, 135.0167) -> (-0.0373, 132.5167)
  line L1643 (-0.0373, 132.5167) -> (-0.0373, 127.5167)
  line L1644 (-0.0373, 127.5167) -> (4.2929, 125.0167)
  line L1645 (4.2929, 125.0167) -> (8.623, 127.5167)
  line L1646 (8.623, 127.5167) -> (8.623, 132.5167)
  line L1647 (8.623, 132.5167) -> (4.2929, 135.0167)
  line L1648 (14.9531, 135.0167) -> (10.623, 132.5167)
  line L1649 (10.623, 132.5167) -> (10.623, 127.5167)
  line L1650 (10.623, 127.5167) -> (14.9531, 125.0167)
  line L1651 (14.9531, 125.0167) -> (19.2832, 127.5167)
  line L1652 (19.2832, 127.5167) -> (19.2832, 132.5167)
  line L1653 (19.2832, 132.5167) -> (14.9531, 135.0167)
  line L1654 (25.6134, 135.0167) -> (21.2832, 132.5167)
  line L1655 (21.2832, 132.5167) -> (21.2832, 127.5167)
  line L1656 (21.2832, 127.5167) -> (25.6134, 125.0167)
  line L1657 (25.6134, 125.0167) -> (29.9435, 127.5167)
  line L1658 (29.9435, 127.5167) -> (29.9435, 132.5167)
  line L1659 (29.9435, 132.5167) -> (25.6134, 135.0167)
  line L1660 (36.2736, 135.0167) -> (31.9435, 132.5167)
  line L1661 (31.9435, 132.5167) -> (31.9435, 127.5167)
  line L1662 (31.9435, 127.5167) -> (36.2736, 125.0167)
  line L1663 (36.2736, 125.0167) -> (40.6037, 127.5167)
  line L1664 (40.6037, 127.5167) -> (40.6037, 132.5167)
  line L1665 (40.6037, 132.5167) -> (36.2736, 135.0167)
  line L1666 (46.9339, 135.0167) -> (42.6037, 132.5167)
  line L1667 (42.6037, 132.5167) -> (42.6037, 127.5167)
  line L1668 (42.6037, 127.5167) -> (46.9339, 125.0167)
  line L1669 (46.9339, 125.0167) -> (51.264, 127.5167)
  line L1670 (51.264, 127.5167) -> (51.264, 132.5167)
  line L1671 (51.264, 132.5167) -> (46.9339, 135.0167)
  line L1672 (57.5941, 135.0167) -> (53.264, 132.5167)
  line L1673 (53.264, 132.5167) -> (53.264, 127.5167)
  line L1674 (53.264, 127.5167) -> (57.5941, 125.0167)
  line L1675 (57.5941, 125.0167) -> (61.9242, 127.5167)
  line L1676 (61.9242, 127.5167) -> (61.9242, 132.5167)
  line L1677 (61.9242, 132.5167) -> (57.5941, 135.0167)
  line L1678 (68.2544, 135.0167) -> (63.9242, 132.5167)
  line L1679 (63.9242, 132.5167) -> (63.9242, 127.5167)
  line L1680 (63.9242, 127.5167) -> (68.2544, 125.0167)
  line L1681 (68.2544, 125.0167) -> (72.5845, 127.5167)
  line L1682 (72.5845, 127.5167) -> (72.5845, 132.5167)
  line L1683 (72.5845, 132.5167) -> (68.2544, 135.0167)
  line L1684 (78.9146, 135.0167) -> (74.5845, 132.5167)
  line L1685 (74.5845, 132.5167) -> (74.5845, 127.5167)
  line L1686 (74.5845, 127.5167) -> (78.9146, 125.0167)
  line L1687 (78.9146, 125.0167) -> (83.2448, 127.5167)
  line L1688 (83.2448, 127.5167) -> (83.2448, 132.5167)
  line L1689 (83.2448, 132.5167) -> (78.9146, 135.0167)
  line L1690 (89.5749, 135.0167) -> (85.2448, 132.5167)
  line L1691 (85.2448, 132.5167) -> (85.2448, 127.5167)
  line L1692 (85.2448, 127.5167) -> (89.5749, 125.0167)
  line L1693 (89.5749, 125.0167) -> (93.905, 127.5167)
  line L1694 (93.905, 127.5167) -> (93.905, 132.5167)
  line L1695 (93.905, 132.5167) -> (89.5749, 135.0167)
  line L1696 (100.2351, 135.0167) -> (95.905, 132.5167)
  line L1697 (95.905, 132.5167) -> (95.905, 127.5167)
  line L1698 (95.905, 127.5167) -> (100.2351, 125.0167)
  line L1699 (100.2351, 125.0167) -> (104.5653, 127.5167)
  line L1700 (104.5653, 127.5167) -> (104.5653, 132.5167)
  line L1701 (104.5653, 132.5167) -> (100.2351, 135.0167)
  line L1702 (110.8954, 135.0167) -> (106.5653, 132.5167)
  line L1703 (106.5653, 132.5167) -> (106.5653, 127.5167)
  line L1704 (106.5653, 127.5167) -> (110.8954, 125.0167)
  line L1705 (110.8954, 125.0167) -> (115.2255, 127.5167)
  line L1706 (115.2255, 127.5167) -> (115.2255, 132.5167)
  line L1707 (115.2255, 132.5167) -> (110.8954, 135.0167)
  line L1708 (121.5556, 135.0167) -> (117.2255, 132.5167)
  line L1709 (117.2255, 132.5167) -> (117.2255, 127.5167)
  line L1710 (117.2255, 127.5167) -> (121.5556, 125.0167)
  line L1711 (121.5556, 125.0167) -> (125.8858, 127.5167)
  line L1712 (125.8858, 127.5167) -> (125.8858, 132.5167)
  line L1713 (125.8858, 132.5167) -> (121.5556, 135.0167)
  line L1714 (132.2159, 135.0167) -> (127.8858, 132.5167)
  line L1715 (127.8858, 132.5167) -> (127.8858, 127.5167)
  line L1716 (127.8858, 127.5167) -> (132.2159, 125.0167)
  line L1717 (132.2159, 125.0167) -> (136.546, 127.5167)
  line L1718 (136.546, 127.5167) -> (136.546, 132.5167)
  line L1719 (136.546, 132.5167) -> (132.2159, 135.0167)
  line L1720 (142.8762, 135.0167) -> (138.546, 132.5167)
  line L1721 (138.546, 132.5167) -> (138.546, 127.5167)
  line L1722 (138.546, 127.5167) -> (142.8762, 125.0167)
  line L1723 (142.8762, 125.0167) -> (147.2063, 127.5167)
  line L1724 (147.2063, 127.5167) -> (147.2063, 132.5167)
  line L1725 (147.2063, 132.5167) -> (142.8762, 135.0167)
  line L1726 (-64.9988, 144.2487) -> (-69.3289, 141.7487)
  line L1727 (-69.3289, 141.7487) -> (-69.3289, 136.7487)
  line L1728 (-69.3289, 136.7487) -> (-64.9988, 134.2487)
  line L1729 (-64.9988, 134.2487) -> (-60.6687, 136.7487)
  line L1730 (-60.6687, 136.7487) -> (-60.6687, 141.7487)
  line L1731 (-60.6687, 141.7487) -> (-64.9988, 144.2487)
  line L1732 (-54.3385, 144.2487) -> (-58.6687, 141.7487)
  line L1733 (-58.6687, 141.7487) -> (-58.6687, 136.7487)
  line L1734 (-58.6687, 136.7487) -> (-54.3385, 134.2487)
  line L1735 (-54.3385, 134.2487) -> (-50.0084, 136.7487)
  line L1736 (-50.0084, 136.7487) -> (-50.0084, 141.7487)
  line L1737 (-50.0084, 141.7487) -> (-54.3385, 144.2487)
  line L1738 (-43.6783, 144.2487) -> (-48.0084, 141.7487)
  line L1739 (-48.0084, 141.7487) -> (-48.0084, 136.7487)
  line L1740 (-48.0084, 136.7487) -> (-43.6783, 134.2487)
  line L1741 (-43.6783, 134.2487) -> (-39.3482, 136.7487)
  line L1742 (-39.3482, 136.7487) -> (-39.3482, 141.7487)
  line L1743 (-39.3482, 141.7487) -> (-43.6783, 144.2487)
  line L1744 (-33.018, 144.2487) -> (-37.3482, 141.7487)
  line L1745 (-37.3482, 141.7487) -> (-37.3482, 136.7487)
  line L1746 (-37.3482, 136.7487) -> (-33.018, 134.2487)
  line L1747 (-33.018, 134.2487) -> (-28.6879, 136.7487)
  line L1748 (-28.6879, 136.7487) -> (-28.6879, 141.7487)
  line L1749 (-28.6879, 141.7487) -> (-33.018, 144.2487)
  line L1750 (-22.3578, 144.2487) -> (-26.6879, 141.7487)
  line L1751 (-26.6879, 141.7487) -> (-26.6879, 136.7487)
  line L1752 (-26.6879, 136.7487) -> (-22.3578, 134.2487)
  line L1753 (-22.3578, 134.2487) -> (-18.0277, 136.7487)
  line L1754 (-18.0277, 136.7487) -> (-18.0277, 141.7487)
  line L1755 (-18.0277, 141.7487) -> (-22.3578, 144.2487)
  line L1756 (-11.6975, 144.2487) -> (-16.0277, 141.7487)
  line L1757 (-16.0277, 141.7487) -> (-16.0277, 136.7487)
  line L1758 (-16.0277, 136.7487) -> (-11.6975, 134.2487)
  line L1759 (-11.6975, 134.2487) -> (-7.3674, 136.7487)
  line L1760 (-7.3674, 136.7487) -> (-7.3674, 141.7487)
  line L1761 (-7.3674, 141.7487) -> (-11.6975, 144.2487)
  line L1762 (-1.0373, 144.2487) -> (-5.3674, 141.7487)
  line L1763 (-5.3674, 141.7487) -> (-5.3674, 136.7487)
  line L1764 (-5.3674, 136.7487) -> (-1.0373, 134.2487)
  line L1765 (-1.0373, 134.2487) -> (3.2929, 136.7487)
  line L1766 (3.2929, 136.7487) -> (3.2929, 141.7487)
  line L1767 (3.2929, 141.7487) -> (-1.0373, 144.2487)
  line L1768 (9.623, 144.2487) -> (5.2929, 141.7487)
  line L1769 (5.2929, 141.7487) -> (5.2929, 136.7487)
  line L1770 (5.2929, 136.7487) -> (9.623, 134.2487)
  line L1771 (9.623, 134.2487) -> (13.9531, 136.7487)
  line L1772 (13.9531, 136.7487) -> (13.9531, 141.7487)
  line L1773 (13.9531, 141.7487) -> (9.623, 144.2487)
  line L1774 (20.2832, 144.2487) -> (15.9531, 141.7487)
  line L1775 (15.9531, 141.7487) -> (15.9531, 136.7487)
  line L1776 (15.9531, 136.7487) -> (20.2832, 134.2487)
  line L1777 (20.2832, 134.2487) -> (24.6134, 136.7487)
  line L1778 (24.6134, 136.7487) -> (24.6134, 141.7487)
  line L1779 (24.6134, 141.7487) -> (20.2832, 144.2487)
  line L1780 (30.9435, 144.2487) -> (26.6134, 141.7487)
  line L1781 (26.6134, 141.7487) -> (26.6134, 136.7487)
  line L1782 (26.6134, 136.7487) -> (30.9435, 134.2487)
  line L1783 (30.9435, 134.2487) -> (35.2736, 136.7487)
  line L1784 (35.2736, 136.7487) -> (35.2736, 141.7487)
  line L1785 (35.2736, 141.7487) -> (30.9435, 144.2487)
  line L1786 (41.6037, 144.2487) -> (37.2736, 141.7487)
  line L1787 (37.2736, 141.7487) -> (37.2736, 136.7487)
  line L1788 (37.2736, 136.7487) -> (41.6037, 134.2487)
  line L1789 (41.6037, 134.2487) -> (45.9339, 136.7487)
  line L1790 (45.9339, 136.7487) -> (45.9339, 141.7487)
  line L1791 (45.9339, 141.7487) -> (41.6037, 144.2487)
  line L1792 (52.264, 144.2487) -> (47.9339, 141.7487)
  line L1793 (47.9339, 141.7487) -> (47.9339, 136.7487)
  line L1794 (47.9339, 136.7487) -> (52.264, 134.2487)
  line L1795 (52.264, 134.2487) -> (56.5941, 136.7487)
  line L1796 (56.5941, 136.7487) -> (56.5941, 141.7487)
  line L1797 (56.5941, 141.7487) -> (52.264, 144.2487)
  line L1798 (62.9242, 144.2487) -> (58.5941, 141.7487)
  line L1799 (58.5941, 141.7487) -> (58.5941, 136.7487)
  line L1800 (58.5941, 136.7487) -> (62.9242, 134.2487)
  line L1801 (62.9242, 134.2487) -> (67.2544, 136.7487)
  line L1802 (67.2544, 136.7487) -> (67.2544, 141.7487)
  line L1803 (67.2544, 141.7487) -> (62.9242, 144.2487)
  line L1804 (73.5845, 144.2487) -> (69.2544, 141.7487)
  line L1805 (69.2544, 141.7487) -> (69.2544, 136.7487)
  line L1806 (69.2544, 136.7487) -> (73.5845, 134.2487)
  line L1807 (73.5845, 134.2487) -> (77.9146, 136.7487)
  line L1808 (77.9146, 136.7487) -> (77.9146, 141.7487)
  line L1809 (77.9146, 141.7487) -> (73.5845, 144.2487)
  line L1810 (84.2448, 144.2487) -> (79.9146, 141.7487)
  line L1811 (79.9146, 141.7487) -> (79.9146, 136.7487)
  line L1812 (79.9146, 136.7487) -> (84.2448, 134.2487)
  line L1813 (84.2448, 134.2487) -> (88.5749, 136.7487)
  line L1814 (88.5749, 136.7487) -> (88.5749, 141.7487)
  line L1815 (88.5749, 141.7487) -> (84.2448, 144.2487)
  line L1816 (94.905, 144.2487) -> (90.5749, 141.7487)
  line L1817 (90.5749, 141.7487) -> (90.5749, 136.7487)
  line L1818 (90.5749, 136.7487) -> (94.905, 134.2487)
  line L1819 (94.905, 134.2487) -> (99.2351, 136.7487)
  line L1820 (99.2351, 136.7487) -> (99.2351, 141.7487)
  line L1821 (99.2351, 141.7487) -> (94.905, 144.2487)
  line L1822 (105.5653, 144.2487) -> (101.2351, 141.7487)
  line L1823 (101.2351, 141.7487) -> (101.2351, 136.7487)
  line L1824 (101.2351, 136.7487) -> (105.5653, 134.2487)
  line L1825 (105.5653, 134.2487) -> (109.8954, 136.7487)
  line L1826 (109.8954, 136.7487) -> (109.8954, 141.7487)
  line L1827 (109.8954, 141.7487) -> (105.5653, 144.2487)
  line L1828 (116.2255, 144.2487) -> (111.8954, 141.7487)
  line L1829 (111.8954, 141.7487) -> (111.8954, 136.7487)
  line L1830 (111.8954, 136.7487) -> (116.2255, 134.2487)
  line L1831 (116.2255, 134.2487) -> (120.5556, 136.7487)
  line L1832 (120.5556, 136.7487) -> (120.5556, 141.7487)
  line L1833 (120.5556, 141.7487) -> (116.2255, 144.2487)
  line L1834 (126.8858, 144.2487) -> (122.5556, 141.7487)
  line L1835 (122.5556, 141.7487) -> (122.5556, 136.7487)
  line L1836 (122.5556, 136.7487) -> (126.8858, 134.2487)
  line L1837 (126.8858, 134.2487) -> (131.2159, 136.7487)
  line L1838 (131.2159, 136.7487) -> (131.2159, 141.7487)
  line L1839 (131.2159, 141.7487) -> (126.8858, 144.2487)
  line L1840 (137.546, 144.2487) -> (133.2159, 141.7487)
  line L1841 (133.2159, 141.7487) -> (133.2159, 136.7487)
  line L1842 (133.2159, 136.7487) -> (137.546, 134.2487)